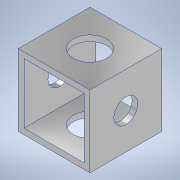
# Autodesk Inventor part: ロボットベース15x15x15
Saved by Autodesk Inventor 2020.3 (Build 243373000, 373)
## iProperties
Created: 2020-07-04
Part Number: ロボットベース15x15x15
Material: アルミニウム 6061
Document SubType Name: Modeling
Designer: totot
Density: 2.7 g/cm^3
Appearance: アルミニウム - フラット
Mass: 2.30611 g
Surface Area: 16.4648 cm^2
Volume: 0.854113 cm^3
Author: totot
Autodesk Inventor part; units mm, degrees
ref_plane "YZ Plane" through (0, 0, 0) normal (1, 0, 0) x (0, 1, 0)
ref_plane "XZ Plane" through (0, 0, 0) normal (0, 1, 0) x (-1, 0, 0)
ref_plane "XY Plane" through (0, 0, 0) normal (0, 0, 1) x (1, 0, 0)
sketch "スケッチ1" plane through (0, 0, 0) normal (0, 0, 1) x (1, 0, 0)
  line L0 (0, 0) -> (-15, 0)
  line L1 (-15, 0) -> (-15, -15)
  line L2 (-15, -15) -> (0, -15)
  line L3 (0, -15) -> (0, 0)
  line L4 (-13.8, -1.2) -> (-1.2, -1.2)
  line L5 (-1.2, -1.2) -> (-1.2, -13.8)
  line L6 (-1.2, -13.8) -> (-13.8, -13.8)
  line L7 (-13.8, -13.8) -> (-13.8, -1.2)
  dimension "d0" = 15
  dimension "d1" = 15
  dimension "d2" = 1.2
  dimension "d3" = 1.2
  dimension "d4" = 1.2
  dimension "d5" = 1.2
  constraints: 16 end point, 4 parallel, 2 horizontal, 2 perpendicular
  measures "d0" distance of L2.end L1.end
  measures "d1" distance of L1.end L0.end
  measures "d2" distance between parallel lines of L1 L7
  measures "d3" distance between parallel lines of L4 L0
  measures "d4" distance between parallel lines of L3 L5
  measures "d5" distance between parallel lines of L2 L6
extrude "押し出し1" add sketch "スケッチ1" along normal blind 15
sketch "スケッチ2" plane through (0, -15, 0) normal (1, 0, 0) x (0, 0, -1)
  line L0 (-15, 0) -> (-15, 15) projected
  line L1 (0, 15) -> (-15, 15) projected
  point P0 (-7.5, 7.5)
  dimension "d8" = 7.5
  dimension "d9" = 7.5
  measures "d8" distance from line of point (-7.5, 7.5) L0
  measures "d9" distance from line of point (-7.5, 7.5) L1
hole "穴1" at (0, -7.5, 7.5) direction (-1, 0, 0) diameter 5 end through all
sketch "スケッチ3" plane through (-15, -15, 0) normal (0, -1, 0) x (1, 0, 0)
  line L0 (0, 0) -> (15, 0) projected
  line L1 (0, 0) -> (0, 15) projected
  point P0 (7.5, 7.5)
  dimension "d17" = 7.5
  dimension "d18" = 7.5
  measures "d17" distance from line of point (7.5, 7.5) L0
  measures "d18" distance from line of point (7.5, 7.5) L1
hole "穴2" at (-7.5, -15, 7.5) direction (0, 1, 0) diameter 7 end through all
equation "\"d3\" = d2"
equation "\"d4\" = d3"
equation "\"d5\" = d3"
equation "\"d9\" = d8"
equation "\"d18\" = d17"
